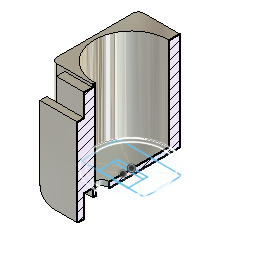
Beacon (Autodesk Fusion 360 design; units mm, degrees)
Autodesk Fusion 360 part; units mm, degrees
sketch "Sketch1" plane through (0, 0, 0) normal (0, 0, 1) x (1, 0, 0)
  circle A0 centre (0, 0) radius 13.5
  circle A1 centre (0, 0) radius 11.75
  line L0 (-11.613, 6.8839) -> (11.613, 6.8839)
  line L1 (11.613, 6.8839) -> (11.613, -6.8839)
  line L2 (11.613, -6.8839) -> (-11.613, -6.8839)
  line L3 (-11.613, -6.8839) -> (-11.613, 6.8839)
  line L4 (-11.613, 6.8839) -> (11.613, -6.8839) construction
  line L5 (11.613, 6.8839) -> (-11.613, -6.8839) construction
  line L6 (5.6708, 0.1161) -> (-5.3292, 0.1161)
  line L7 (-5.3292, 0.1161) -> (-5.3292, -6.8839)
  line L8 (-5.3292, -6.8839) -> (5.6708, -6.8839)
  line L9 (5.6708, -6.8839) -> (5.6708, 0.1161)
  line L10 (5.6708, 0.1161) -> (-5.3292, -6.8839) construction
  line L11 (-5.3292, 0.1161) -> (5.6708, -6.8839) construction
  line L12 (-5.3292, -1.3839) -> (5.6708, -1.3839)
  circle A2 centre (0, 0) radius 13.575
  point P0 (0.1708, -3.3839)
  dimension "d1" = 27
  dimension "d4" = 23.5
  dimension "d9" = 11
  dimension "d10" = 7
  dimension "d14" = 1.5
  dimension "d71" = 27.15
  constraint coincident A0.centre A1.centre
  constraint concentric A0 A1
  constraint horizontal L0
  constraint perpendicular L0 L1
  constraint parallel L0 L2
  constraint parallel L1 L3
  constraint coincident L4 A0.centre
  constraint coincident L5 A0.centre
  constraint coincident A0 L0.start
  constraint horizontal L6
  constraint perpendicular L6 L7
  constraint parallel L6 L8
  constraint parallel L7 L9
  constraint coincident L10 P0
  constraint coincident L11 P0
  constraint collinear L2 L8
  constraint coincident L7 L12.start
  constraint coincident L9 L12.end
  constraint perpendicular L9 L12
  measures "d1" diameter of A0
  measures "d4" diameter of A1
  measures "d9" distance of L7.end L8.end
  measures "d10" distance of L6.end L7.end
  measures "d14" distance of L6 L12
  measures "d71" diameter of A2
extrude "Extrude1" add sketch "Sketch1" along normal blind 190 contours A0 A1 L1 | A0 A1 L0 | A1 L0 L1 | A1 L1 L2 | A0 A1 L2 | A0 A1 L3 | A1 L0 L3 | A1 L0 | A1 L0 L1 L2 L3 L6 L7 L9 | A1 L1 | A1 L2 L3 | A1 L2 L8 | A1 L3 | L2 L7 L8 L9 L12 | L6 L7 L9 L12 makes body 1
extrude "Extrude2" cut sketch "Sketch1" along normal blind 264.214 contours A1 L0 | A1 L0 L1 L2 L3 L6 L7 L9 | A1 L1 | A1 L2 L8 | A1 L3 | L2 L7 L8 L9 L12 | L6 L7 L9 L12 bodies 1
extrude "Extrude3" add sketch "Sketch1" along normal blind 1.5 separate body contours A1 L0 L1 L2 L3 L6 L7 L9 makes body 2
sphere "SpherePrimitive1" add diameter 26.8964 placed x (-1, 0, 0) y (0, -1, 0) z (0, 0, 1) at (0, 0, 190) bodies 1 2
extrude "Extrude4" add sketch "Sketch1" along normal blind 180 contours L6 L7 L9 L12 bodies 2
extrude "Extrude5" add sketch "Sketch1" along normal blind 190 and the other way blind -178.5 contours A1 L0 L1 L2 L3 L6 L7 L9 bodies 1 2
ref_plane "WorkPlane1" through (0, 0, 180) normal (0, 0, 1) x (1, 0, 0)
sketch "Sketch3" plane through (0, 0, 180) normal (0, 0, 1) x (1, 0, 0)
sphere "SpherePrimitive2" cut diameter 23.5 placed x (1, 0, 0) y (0, 1, 0) z (0, 0, 1) at (0, 0, 180) bodies 1
extrude "Extrude6" cut sketch "Sketch1" along normal blind 180 contours A1 L0 | A1 L0 L1 L2 L3 L6 L7 L9 | A1 L1 | A1 L2 L8 | A1 L3 | L2 L7 L8 L9 L12 | L6 L7 L9 L12 bodies 1
sketch "Sketch6" plane through (0, -1.3839, 0) normal (0, -1, 0) x (1, 0, 0)
ref_plane "WorkPlane2" through (0.1708, -12.4989, 90) normal (0, -1, 0) x (1, 0, 0)
sketch "Sketch7" plane through (0, -12.4989, 0) normal (0, -1, 0) x (-1, 0, 0)
  line L0 (-13, 0) -> (13, 0)
  line L1 (13, 0) -> (13, -34)
  line L2 (13, -34) -> (-13, -34)
  line L3 (-13, -34) -> (-13, 0)
  line L4 (13, -34) -> (-13, 0) construction
  line L5 (-13, -34) -> (13, 0) construction
  line L6 (-10, -1) -> (10, -1)
  line L7 (10, -1) -> (10, -33)
  line L8 (10, -33) -> (-10, -33)
  line L9 (-10, -33) -> (-10, -1)
  line L10 (-10, -1) -> (10, -33) construction
  line L11 (10, -1) -> (-10, -33) construction
  point P0 (0, -17)
  dimension "d27" = 26
  dimension "d28" = 34
  dimension "d29" = 13
  dimension "d30" = 20
  dimension "d31" = 32
  constraint horizontal L0
  constraint vertical L1
  constraint horizontal L2
  constraint vertical L3
  constraint horizontal L6
  constraint perpendicular L6 L7
  constraint parallel L6 L8
  constraint parallel L7 L9
  constraint coincident L10 P0
  constraint coincident L11 P0
  constraint midpoint L5 P0
  measures "d27" distance of L0.start L0.end
  measures "d28" distance of L0.start L2.end
  measures "d29" distance of L3 origin
  measures "d30" distance of L7.end L8.end
  measures "d31" distance of L6.end L7.end
extrude "Extrude7" add sketch "Sketch7" along normal blind 2 bodies 1
extrude "Extrude8" add sketch "Sketch7" along normal blind 5.1 contours L6 L7 L8 L9 bodies 1
sketch "Sketch8" plane through (0, -17.5989, 0) normal (0, -1, 0) x (1, 0, 0)
  line L0 (10, 33) -> (-10, 33)
  line L1 (-10, 33) -> (-10, 1)
  line L2 (-10, 1) -> (10, 1)
  line L3 (10, 1) -> (10, 33)
  line L4 (-10, 24.8231) -> (10, 24.8231)
  line L5 (10, 24.8231) -> (10, -7.1769)
  line L6 (10, -7.1769) -> (-10, -7.1769)
  line L7 (-10, -7.1769) -> (-10, 24.8231)
  dimension "d36" = 32
  constraint horizontal L4
  constraint vertical L5
  constraint horizontal L6
  constraint vertical L7
  constraint coincident L1 L4.start
  measures "d36" distance of L4.start L6.end
extrude "Extrude9" add sketch "Sketch8" along normal blind 2.5 contours L1 L2 L3 L4 L5 L7 | L2 L5 L6 L7 bodies 1
sketch "Sketch9" plane through (10, 0, 0) normal (1, 0, 0) x (0, 1, 0)
  line L0 (-14.4989, 1) -> (-14.4989, 33)
  line L1 (-14.4989, 33) -> (-17.5989, 33)
  line L2 (-17.5989, 33) -> (-17.5989, 24.8231)
  line L3 (-17.5989, 24.8231) -> (-20.0989, 24.8231)
  line L4 (-20.0989, 24.8231) -> (-20.0989, -7.1769)
  line L5 (-20.0989, -7.1769) -> (-17.5989, -7.1769)
  line L6 (-17.5989, -7.1769) -> (-17.5989, 1)
  line L7 (-17.5989, 1) -> (-14.4989, 1)
  line L8 (-20.0989, 24.8231) -> (-17.5989, 24.8231)
  line L9 (-17.5989, 24.8231) -> (-17.5989, -7.1769)
  line L10 (-17.5989, -7.1769) -> (-20.0989, -7.1769)
  line L11 (-20.0989, -7.1769) -> (-20.0989, 24.8231)
  constraint horizontal L8
  constraint vertical L9
  constraint horizontal L10
  constraint vertical L11
  constraint coincident L5.end L6.start
  constraint coincident L3.end L4.start
extrude "Extrude12" add sketch "Sketch9" along normal blind 3.25 contours L3 L4 L5 L6 L8 L9 L10 L11 bodies 1
extrude "Extrude13" add sketch "Sketch9" along normal blind -23.5 and the other way blind 20 contours L3 L4 L5 L6 L8 L9 L10 L11 bodies 1
extrude "Extrude10" add 2 faces at (7.7345, -12.4989, 22.6667) (-7.7345, -12.4989, 22.6667) along direction (0, 1, 0) blind 11.872 on bodies 1 bodies 1
extrude "Extrude11" cut sketch "Sketch1" along normal blind 34 contours A1 L0 L1 L2 L3 L6 L7 L9 | A1 L1 | A1 L2 L8 | A1 L3 | L2 L7 L8 L9 L12 | L6 L7 L9 L12 bodies 1
fillet "Fillet2" radius 5 2 edges at (13.25, -18.8489, -7.1769) (-13.5, -18.8489, -7.1769) on bodies 1
extrude "Extrude14" add 1 faces at (13, -10.8793, 11.3333) along direction (1, 0, 0) blind 2 on bodies 1 bodies 1
extrude "Extrude15" add 1 faces at (-13, -10.8793, 22.6667) along direction (-1, 0, 0) blind 2 on bodies 1 bodies 1
extrude "Extrude16" cut sketch "Sketch1" along normal blind 34 contours A0 A1 L1 | A0 A1 L0 | A1 L0 L1 | A1 L1 L2 | A0 A1 L2 | A0 A1 L3 | A1 L0 L3 | A1 L2 L3 bodies 1
extrude "Extrude17" add sketch "Sketch7" against normal blind 30 contours L0 L1 L2 L3 | L6 L7 L8 L9 bodies 1
extrude "Extrude18" add 1 faces at (-14.3333, -3.6401, 22.6667) along direction (0, 1, 0) blind 21.141 on bodies 1 bodies 1
extrude "Extrude19" add 1 faces at (13.6667, -3.6401, 22.6667) along direction (0, 1, 0) blind 21.141 on bodies 1 bodies 1
split "Split1" by plane through (13, -3.6401, 34) normal (0, 0, 1) bodies 1 makes body 3 at (0, -13.5, 138)
extrude "Extrude20" cut sketch "Sketch1" along normal blind 34 contours A0 A1 L1 | A0 A1 L0 | A1 L0 L1 | A1 L1 L2 | A0 A1 L2 | A0 A1 L3 | A1 L0 L3 | A1 L0 | A1 L0 L1 L2 L3 L6 L7 L9 | A1 L1 | A1 L2 L3 | A1 L2 L8 | A1 L3 | L2 L7 L8 L9 L12 | L6 L7 L9 L12 | A2 bodies 1
extrude "Extrude21" add 2 faces at (-1.1497, -12.6833, 34) (-5.9596, -11.4256, 34) along direction (0, 0, -1) blind 34 on bodies 3 bodies 3
sketch "Sketch10" plane through (0, 0, 0) normal (0, 0, -1) x (1, 0, 0)
  circle A0 centre (0, 0) radius 13.575
  line L0 (-13, -17.5009) -> (-13, -17.5011)
  line L1 (-13, -17.5011) -> (13, -17.5011)
  line L2 (13, -17.5011) -> (13, -17.5009)
  line L3 (13, -17.5009) -> (15, -17.5009)
  line L4 (15, -17.5009) -> (15, 14.4989)
  line L5 (15, 14.4989) -> (-15, 14.4989)
  line L6 (-15, 14.4989) -> (-15, -17.5009)
  line L7 (-15, -17.5009) -> (-13, -17.5009)
  line L8 (15, -17.5009) -> (-15, -17.5009)
  line L9 (-15, -17.5009) -> (-15, 14.4989)
  line L10 (-15, 14.4989) -> (15, 14.4989)
  line L11 (15, 14.4989) -> (15, -17.5009)
  circle A1 centre (0, 10.8) radius 2.5
  dimension "d76" = 5
  constraint horizontal L8
  constraint vertical L9
  constraint horizontal L10
  constraint vertical L11
  constraint coincident L5.end L6.start
  constraint coincident L3.end L4.start
  measures "d76" diameter of A1
extrude "Extrude22" add sketch "Sketch10" along normal blind 2 contours A0 | L1 L3 L4 L5 L6 L7 L8 L9 L10 L11 bodies 1
fillet "Fillet5" radius 2 4 edges at (-15, -14.4989, 16) (-15, 17.5009, 16) (15, -14.4989, 16) (15, 17.5009, 16) on bodies 1
extrude "Extrude23" cut sketch "Sketch1" along normal blind 190.376 contours A1 L0 | A1 L0 L1 L2 L3 L6 L7 L9 | A1 L2 L8 | L2 L7 L8 L9 L12 | L6 L7 L9 L12 bodies 3
sphere "SpherePrimitive4" cut diameter 23.46 placed x (1, 0, 0) y (0, -1, 0) z (0, 0, -1) at (0, 0, 190.376) bodies 3
extrude "Extrude24" add sketch "Sketch1" along normal blind 190.283 and the other way blind -189 separate body contours A1 L0 L1 L2 L3 L6 L7 L9 | L6 L7 L9 L12 makes body 4
extrude "Extrude25" add sketch "Sketch1" along normal blind 1.5 separate body contours A1 L0 L1 L2 L3 L6 L7 L9 | L6 L7 L9 L12 makes body 5
extrude "Extrude26" add sketch "Sketch1" along normal blind 190.283 contours L6 L7 L9 L12 bodies 4 5
hidden bodies 3 4
named bodies: "Tube Holder", "LED holder", "Tube (1)", "Led Holder"
